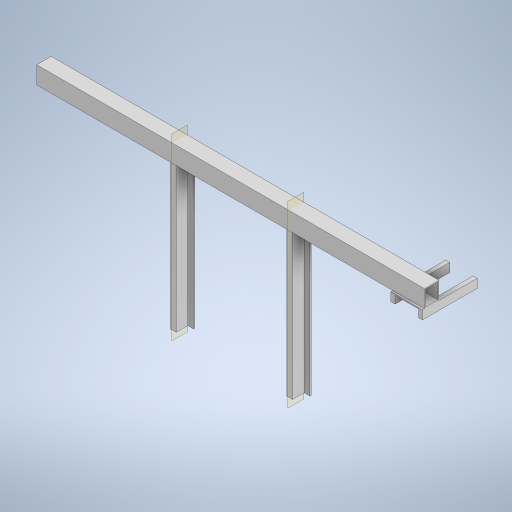
# Autodesk Inventor part: Trave_e_Pale_inventor_single
Saved by Autodesk Inventor 2024.2 (Build 282272000, 272)
## iProperties
Created: 2024-03-18
Part Number: Trave_e_Pale_inventor_single
Material: Generic
Document SubType Name: Modeling
Designer: feder
Density: 1 g/cm^3
Appearance: Default
Author: feder
Autodesk Inventor part; units mm, degrees
ref_plane "YZ Plane" through (0, 0, 0) normal (1, 0, 0) x (0, 1, 0)
ref_plane "XZ Plane" through (0, 0, 0) normal (0, 1, 0) x (-1, 0, 0)
ref_plane "XY Plane" through (0, 0, 0) normal (0, 0, 1) x (1, 0, 0)
sketch "Sketch1" plane through (0, 0, 0) normal (0, 1, 0) x (-1, 0, 0)
  line L0 (0, 0) -> (-1400, 0) construction
  line L1 (-1400, 0) -> (-2600, 0) construction
  line L2 (-2600, 0) -> (-4000, 0) construction
  line L3 (-4000, 75) -> (0, 75)
  line L4 (0, 75) -> (0, -75)
  line L5 (0, -75) -> (-4000, -75)
  line L6 (-4000, -75) -> (-4000, 75)
  line L7 (-4000, 75) -> (0, -75) construction
  line L8 (0, 75) -> (-4000, -75) construction
  point P0 (-2000, 0)
  dimension "d0" = 1400
  dimension "d1" = 1200
  dimension "d2" = 1400
  dimension "d3" = 150
  dimension "d4" = 4000
  constraints: 18 end point, 3 midpoint, 3 parallel, 2 point on line, 1 horizontal, 1 perpendicular
  measures "d0" distance of L0.start L0.end
  measures "d1" distance of L0.end L1.end
  measures "d2" distance of L1.end L2.end
  measures "d3" distance of L3.end L4.end
  measures "d4" distance between parallel lines of L6 L4
extrude "Extrusion1" add sketch "Sketch1" along normal blind 180
shell "Shell1" thickness 10 removed faces 2 at (0, 60, -25) at (4000, 60, 25)
sketch "Sketch2" plane through (0, 0, 0) normal (0, -1, 0) x (1, 0, 0)
  line L0 (0, 0) -> (1400, 0) construction
  line L1 (1400, 0) -> (2600, 0) construction
  line L2 (2600, 0) -> (4000, 0) construction
  line L3 (0, -75) -> (0, 75) construction
  line L4 (4000, 75) -> (4000, -75) construction
  line L5 (0, 75) -> (4000, 75) construction
  line L6 (4000, 75) -> (4000, -75) construction
  line L7 (4000, -75) -> (0, -75) construction
  line L8 (0, -75) -> (0, 75) construction
  line L9 (3991, 66) -> (9, 66) construction
  line L10 (9, 66) -> (9, -66) construction
  line L11 (9, -66) -> (3991, -66) construction
  line L12 (3991, -66) -> (3991, 66) construction
  line L13 (1370, -66) -> (1370, 66) construction
  line L14 (1370, 66) -> (1430, 66) construction
  line L15 (1430, 66) -> (1430, -66) construction
  line L16 (1430, -66) -> (1370, -66) construction
  line L17 (1370, -66) -> (1430, 66) construction
  line L18 (1370, 66) -> (1430, -66) construction
  line L19 (1310, -66) -> (1310, 66) construction
  line L20 (1310, 66) -> (1490, 66) construction
  line L21 (1490, 66) -> (1490, -66) construction
  line L22 (1490, -66) -> (1310, -66) construction
  line L23 (1310, -66) -> (1490, 66) construction
  line L24 (1310, 66) -> (1490, -66) construction
  line L25 (1310, -66) -> (1490, -66) construction
  line L26 (1490, -66) -> (1490, -54) construction
  line L27 (1490, -54) -> (1310, -54) construction
  line L28 (1310, -54) -> (1310, -66) construction
  line L29 (1370, -54) -> (1430, -54) construction
  line L30 (1430, -54) -> (1430, 66) construction
  line L31 (1430, 66) -> (1370, 66) construction
  line L32 (1370, 66) -> (1370, -54) construction
  line L33 (1310, -54) -> (1370, -54)
  line L34 (1370, 66) -> (1370, -54)
  line L35 (1430, -54) -> (1430, 66)
  line L36 (1370, 66) -> (1430, 66)
  line L37 (1430, -54) -> (1490, -54)
  line L38 (1310, -54) -> (1310, -66)
  line L39 (1310, -66) -> (1490, -66)
  line L40 (1490, -54) -> (1490, -66)
  line L41 (4000, -65) -> (0, -65) projected
  line L42 (1376, -54) -> (1376, 60)
  line L43 (1376, 60) -> (1424, 60)
  line L44 (1424, 60) -> (1424, -54)
  line L45 (1376, -54) -> (1424, -54)
  point P0 (1310, -65)
  point P1 (1490, -65)
  dimension "d8" = 1400
  dimension "d9" = 1200
  dimension "d10" = 1400
  dimension "d11" = 9
  dimension "d12" = 60
  dimension "d13" = 180
  dimension "d14" = 12
  dimension "d15" = 6
  dimension "d16" = 114
  constraints: 86 end point, 13 parallel, 9 perpendicular, 7 point on line, 6 collinear, 4 horizontal, 4 midpoint, 3 other
  measures "d8" distance of L0.start L0.end
  measures "d9" distance of L0.end L1.end
  measures "d10" distance of L1.end L2.end
  measures "d11" distance between parallel lines of L5 L9
  measures "d12" distance of L13.end L14.end
  measures "d13" distance of L19.end L20.end
  measures "d14" distance of L26.end L25.end
  measures "d15" distance between parallel lines of L32 L42
  measures "d16" distance between parallel lines of L27 L43
extrude "Extrusion2" add sketch "Sketch2" along normal blind 1500 contours L33 L34 L36 L35 L37 L40 L41 L38
ref_plane "Work Plane1" through (1400, -1500, -54) normal (1, 0, 0) x (0, 0, -1)
ref_plane "Work Plane3" through (2000, -1500, -54) normal (1, 0, 0) x (0, 0, -1)
ref_plane "Work Plane2" through (2600, -1500, -54) normal (1, 0, 0) x (0, 0, -1)
mirror "Mirror1" about plane through (2000, -1500, -54) normal (1, 0, 0) of "Extrusion2"
sketch "Sketch3" plane through (0, 0, 75) normal (0, 0, 1) x (1, 0, 0)
  line L0 (4000, 0) -> (0, 0) projected
  line L1 (4000, 0) -> (3675, 0)
  line L2 (3675, 0) -> (3675, -90)
  line L3 (3675, -90) -> (4000, -90)
  line L4 (4000, -90) -> (4000, 0)
  line L5 (3675, 0) -> (3717.5, 0)
  line L6 (3717.5, 0) -> (3717.5, -90)
  line L7 (3717.5, -90) -> (3675, -90)
  line L8 (3675, -90) -> (3675, 0)
  line L9 (4000, -90) -> (3957.5, -90)
  line L10 (3957.5, -90) -> (3957.5, 0)
  line L11 (3957.5, 0) -> (4000, 0)
  line L12 (4000, 0) -> (4000, -90)
  line L13 (3717.5, 0) -> (3957.5, 0)
  line L14 (3957.5, 0) -> (3957.5, -12)
  line L15 (3957.5, -12) -> (3717.5, -12)
  line L16 (3717.5, -12) -> (3717.5, 0)
  dimension "d20" = 325
  dimension "d21" = 90
  dimension "d22" = 42.5
  dimension "d23" = 42.5
  dimension "d24" = 90
  dimension "d25" = 12
  constraints: 32 end point, 8 parallel, 4 horizontal, 4 perpendicular, 2 point on line
  measures "d20" distance of L3.end L2.end
  measures "d21" distance of L2.end L1.end
  measures "d22" distance of L6.end L7.end
  measures "d23" distance of L10.end L11.end
  measures "d24" distance of L9.end L10.end
  measures "d25" distance of L13.end L14.end
extrude "Extrusion3" add sketch "Sketch3" along normal blind 20 and the other way blind 150 contours L4 L3 L10 L0 | L10 L15 L6 L0 | L6 L3 L2 L0
sketch "Sketch5" plane through (4000, 180, -75) normal (0, 0, -1) x (-1, 0, 0)
  line L0 (0, 0) -> (0, -270) projected
  line L1 (0, -270) -> (42.5, -270)
  line L2 (42.5, -270) -> (42.5, -180)
  line L3 (42.5, -180) -> (0, -180)
  line L4 (0, -180) -> (0, -270)
  line L5 (282.5, -270) -> (325, -270) projected
  line L6 (325, -270) -> (282.5, -270)
  line L7 (282.5, -270) -> (282.5, -180)
  line L8 (282.5, -180) -> (325, -180)
  line L9 (325, -180) -> (325, -270)
  point P0 (4000, -180)
  dimension "d36" = 90
  dimension "d37" = 42.5
  dimension "d38" = 90
  constraints: 16 end point, 4 parallel, 2 horizontal, 2 perpendicular
  measures "d36" distance of L2.end L1.end
  measures "d37" distance of L7.end L8.end
  measures "d38" distance of L6.end L7.end
extrude "Extrusion4" add sketch "Sketch5" along normal blind 395
body "Solid1"
